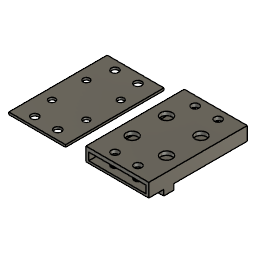
CNC Z axis (Autodesk Fusion 360 design; units mm, degrees)
part number: 2025-09-05-01-01-18-360
Autodesk Fusion 360 part; units mm, degrees
note: some values were not read from the file. Set by a fixed rule: which face or edge a step refers to.
other "Base Mesh Feature1"
other "Modify1"
sketch "Sketch1" plane through (0, 0, 0) normal (0, 0, 1) x (1, 0, 0)
  line L0 (27.5, -43) -> (-27.5, -43)
  line L1 (-27.5, -43) -> (-27.5, 43)
  line L2 (-27.5, 43) -> (27.5, 43)
  line L3 (27.5, 43) -> (27.5, -43)
  line L4 (27.5, -43) -> (-27.5, 43) construction
  line L5 (-27.5, -43) -> (27.5, 43) construction
  circle A0 centre (15, -15) radius 2.8284
  circle A1 centre (15, 15) radius 2.8284
  circle A2 centre (-15, -15) radius 2.8284
  circle A3 centre (-15, 15) radius 2.8284
  circle A4 centre (10, -35) radius 3.25
  circle A5 centre (-10, -35) radius 3.25
  circle A6 centre (10, 35) radius 3.25
  circle A7 centre (-10, 35) radius 3.25
  circle A8 centre (15, -15) radius 4.75
  circle A9 centre (15, 15) radius 4.75
  circle A10 centre (-15, -15) radius 4.75
  circle A11 centre (-15, 15) radius 4.75
  circle A12 centre (3.9244, 36.95) radius 1
  circle A13 centre (-4.0755, 36.95) radius 1
  line L6 (27.5, -21) -> (-27.5, -21)
  line L7 (27.5, 21) -> (-27.5, 21)
  line L8 (27.5, -30) -> (-27.5, -30)
  line L9 (27.5, 30) -> (-27.5, 30)
  line L10 (-6, 30) -> (-6, 43)
  line L11 (5.9128, 30) -> (5.9128, 43)
  line L12 (11.5, -30) -> (10, -29)
  line L13 (10, -29) -> (8.5, -30)
  line L14 (-8.5, -30) -> (-10, -29)
  line L15 (-10, -29) -> (-11.5, -30)
  line L16 (11.5, 30) -> (10, 29)
  line L17 (10, 29) -> (8.5, 30)
  line L18 (-8.5, 30) -> (-10, 29)
  line L19 (-10, 29) -> (-11.5, 30)
  line L20 (5.9128, 31.7978) -> (5.9175, 31.7978)
  line L21 (5.9175, 31.7978) -> (5.9175, 33.3795)
  line L22 (5.9175, 33.3795) -> (5.9128, 33.3795)
  line L23 (-6, 31.7978) -> (-6.0143, 31.7978)
  line L24 (-6.0143, 31.7978) -> (-6.0143, 33.3598)
  line L25 (-6.0143, 33.3598) -> (-6, 33.3598)
  dimension "d1" = 55
  dimension "d2" = 86
  dimension "d3" = 6.5
  dimension "d4" = 6.5
  dimension "d5" = 6.5
  dimension "d6" = 6.5
  dimension "d7" = 9.5
  dimension "d8" = 9.5
  dimension "d9" = 9.5
  dimension "d10" = 9.5
  dimension "d11" = 20
  dimension "d12" = 20
  dimension "d13" = 70
  dimension "d14" = 70
  dimension "d15" = 17.5
  dimension "d16" = 17.5
  dimension "d18" = 8
  dimension "d19" = 2
  dimension "d20" = 2
  dimension "d33" = 6.05
  dimension "d34" = 6.05
  constraint horizontal L0
  constraint perpendicular L0 L1
  constraint parallel L0 L2
  constraint parallel L1 L3
  constraint coincident L4 origin
  constraint coincident L5 origin
  constraint concentric A0 A8
  constraint concentric A1 A9
  constraint concentric A2 A10
  constraint concentric A3 A11
  constraint coincident L1 L6.end
  constraint perpendicular L1 L6
  constraint coincident L1 L7.end
  constraint perpendicular L1 L7
  constraint coincident L1 L8.end
  constraint perpendicular L1 L8
  constraint coincident L1 L9.end
  constraint perpendicular L1 L9
  constraint coincident L3 L8.start
  constraint coincident L3 L6.start
  constraint coincident L3 L7.start
  constraint coincident L3 L9.start
  constraint coincident L9 L10.start
  constraint coincident L2 L10.end
  constraint perpendicular L2 L10
  constraint coincident L9 L11.start
  constraint coincident L2 L11.end
  constraint perpendicular L2 L11
  constraint coincident L8 L12.start
  constraint coincident L8 L13.end
  constraint coincident L8 L14.start
  constraint coincident L8 L15.end
  constraint coincident L9 L16.start
  constraint parallel L15 L16
  constraint coincident L9 L17.end
  constraint parallel L14 L17
  constraint coincident L9 L18.start
  constraint parallel L16 L18
  constraint coincident L9 L19.end
  constraint parallel L17 L19
  constraint coincident L11 L20.start
  constraint perpendicular L11 L20
  constraint perpendicular L20 L21
  constraint coincident L11 L22.end
  constraint perpendicular L11 L22
  constraint coincident L10 L23.start
  constraint perpendicular L10 L23
  constraint perpendicular L23 L24
  constraint coincident L10 L25.end
  constraint perpendicular L10 L25
  measures "d1" distance of L1.end L2.end
  measures "d2" distance of L0.end L1.end
  measures "d3" diameter of A4
  measures "d4" diameter of A5
  measures "d5" diameter of A6
  measures "d6" diameter of A7
  measures "d7" diameter of A8
  measures "d8" diameter of A9
  measures "d9" diameter of A10
  measures "d10" diameter of A11
  measures "d11" distance of A4.centre A5.centre
  measures "d12" distance of A6.centre A7.centre
  measures "d13" vertical distance of A4.centre A6.centre
  measures "d14" vertical distance of A5.centre A7.centre
  measures "d15" distance of L3 A4.centre
  measures "d16" distance of L3 A6.centre
  measures "d18" distance of L0 A4.centre
  measures "d19" diameter of A12
  measures "d20" diameter of A13
  measures "d33" distance of L2 A12.centre
  measures "d34" distance of L2 A13.centre
extrude "Extrude1" add sketch "Sketch1" along normal blind 20 contours L0 L1 L3 L8 | L1 L3 L6 L8 L12 L13 L14 L15 | L1 L3 L6 L7 | L8 L12 L13 | L8 L14 L15 | L1 L3 L7 L9 L16 L17 L18 L19 | L2 L3 L9 L11 L20 L21 L22 | L1 L2 L9 L10 L23 L24 L25 | L9 L16 L17 | L9 L18 L19 | L2 L9 L10 L11 | L11 L20 L21 L22 | L10 L23 L24 L25 | A8 | A9 | A10 | A11 | A12 | A13 makes body 1
extrude "Extrude2" cut sketch "Sketch1" along normal blind 10 contours L1 L3 L6 L7 | A8 | A9 | A10 | A11 bodies 1
extrude "Extrude3" cut sketch "Sketch1" along normal blind 5 contours L1 L3 L6 L8 L12 L13 L14 L15 | L8 L12 L13 | L8 L14 L15 | L1 L3 L7 L9 L16 L17 L18 L19 | L9 L16 L17 | L9 L18 L19 bodies 1
extrude "Extrude4" cut sketch "Sketch1" along normal blind 7 contours A12 | A13 bodies 1
extrude "Extrude5" cut sketch "Sketch1" along normal blind 5 contours L0 L1 L3 L8 bodies 1
extrude "Extrude6" cut sketch "Sketch1" along normal blind 10 contours L2 L3 L9 L11 L20 L21 L22 | L1 L2 L9 L10 L23 L24 L25 | L11 L20 L21 L22 | L10 L23 L24 L25 bodies 1
sketch "Sketch2" plane through (0, 0, 0) normal (0, 0, 1) x (1, 0, 0)
extrude "Extrude7" cut sketch "Sketch1" along normal blind 10 contours L11 L20 L21 L22 | L10 L23 L24 L25 bodies 1
extrude "Extrude8" cut sketch "Sketch1" along normal blind 10 contours L9 L16 L17 | L9 L18 L19 bodies 1
extrude "Extrude9" cut sketch "Sketch1" along normal blind 10 contours L8 L12 L13 | L8 L14 L15 bodies 1
extrude "Extrude10" cut sketch "Sketch1" along normal blind 10 contours L0 L1 L3 L8 bodies 1
extrude "Extrude11" add 1 faces at (-4.3089, 4.3587, 20) along direction (0, 0, 1) blind 4 on bodies 1 bodies 1
sketch "Sketch3" plane through (0, -43, 0) normal (0, -1, 0) x (1, 0, 0)
  line L0 (-27.5, 10) -> (27.5, 10)
  line L1 (27.5, 10) -> (27.5, 24)
  line L2 (-27.5, 24) -> (-27.5, 10)
  line L3 (-26, 15.4) -> (26, 15.4)
  line L4 (26, 15.4) -> (26, 13.1)
  line L5 (26, 13.1) -> (-26, 13.1)
  line L6 (-26, 13.1) -> (-26, 15.4)
  line L7 (-26, 12.7394) -> (26, 12.7394)
  line L8 (26, 12.7394) -> (26, 10.4394)
  line L9 (26, 10.4394) -> (-26, 10.4394)
  line L10 (-26, 10.4394) -> (-26, 12.7394)
  line L11 (27.5, 24) -> (-27.5, 24)
  line L12 (-26, 18.1) -> (26, 18.1)
  line L13 (26, 18.1) -> (26, 15.8)
  line L14 (26, 15.8) -> (-26, 15.8)
  line L15 (-26, 15.8) -> (-26, 18.1)
  dimension "d61" = 2.3
  dimension "d62" = 2.3
  dimension "d65" = 2.3
  constraint horizontal L3
  constraint vertical L4
  constraint horizontal L5
  constraint vertical L6
  constraint horizontal L7
  constraint vertical L8
  constraint horizontal L9
  constraint vertical L10
  constraint horizontal L12
  constraint vertical L13
  constraint horizontal L14
  constraint vertical L15
  measures "d61" distance of L3.start L5.end
  measures "d62" distance of L7.start L9.end
  measures "d65" distance of L12.start L14.end
extrude "Extrude12" cut sketch "Sketch3" against normal blind 90 contours L3 L4 L5 L6 | L7 L8 L9 L10 bodies 1
extrude "Extrude13" add sketch "Sketch3" against normal blind 86 contours L3 L4 L5 L6 | L7 L8 L9 L10 | L12 L13 L14 L15 bodies 1
extrude "Extrude14" cut 1 faces at (-4.3089, 4.3587, 24) along direction (0, 0, -1) blind 0.6 on bodies 1 bodies 1
sketch "Sketch4" plane through (0, 0, 23.4) normal (0, 0, 1) x (-1, 0, 0)
  circle A0 centre (15, -15) radius 2.8284
  circle A1 centre (-15, 15) radius 2.8284
  circle A2 centre (-15, -15) radius 2.8284
  circle A3 centre (-10, -35) radius 3.25
  circle A4 centre (10, 35) radius 3.25
  circle A5 centre (-10, 35) radius 3.25
  circle A6 centre (15, 15) radius 2.8284
  circle A7 centre (10, -35) radius 3.25
  line L0 (-27.5, -43) -> (27.5, -43)
  line L1 (27.5, -43) -> (27.5, 43)
  line L2 (27.5, 43) -> (-27.5, 43)
  line L3 (-27.5, 43) -> (-27.5, -43)
  circle A8 centre (15, 15) radius 5
  circle A9 centre (-15, 15) radius 5
  circle A10 centre (15, -15) radius 5
  circle A11 centre (-15, -15) radius 5
  dimension "d70" = 10
  dimension "d71" = 10
  dimension "d72" = 10
  dimension "d73" = 10
  constraint concentric A6 A8
  constraint concentric A1 A9
  constraint concentric A0 A10
  constraint concentric A2 A11
  measures "d70" diameter of A8
  measures "d71" diameter of A9
  measures "d72" diameter of A10
  measures "d73" diameter of A11
extrude "Extrude15" cut sketch "Sketch4" against normal blind 6 contours A8 | A9 | A10 | A11 bodies 1
sketch "Sketch6" plane through (0, 0, 15.8) normal (0, 0, -1) x (-1, 0, 0)
  circle A0 centre (15, 15) radius 2.8284
  circle A1 centre (-15, -15) radius 2.8284
  circle A2 centre (-15, 15) radius 2.8284
  circle A3 centre (-10, 35) radius 3.25
  circle A4 centre (10, -35) radius 3.25
  circle A5 centre (-10, -35) radius 3.25
  circle A6 centre (15, -15) radius 2.8284
  circle A7 centre (10, 35) radius 3.25
extrude "Extrude17" add 1 faces at (5.9128, 38.6667, 5) along direction (1, 0, 0) blind 1 on bodies 1 bodies 1
extrude "Extrude18" add 1 faces at (-6, 38.6667, 5) along direction (-1, 0, 0) blind 1 on bodies 1 bodies 1
sketch "Sketch7" plane through (0, -43, 0) normal (0, -1, 0) x (1, 0, 0)
  line L0 (27.5, 23.4) -> (-27.5, 23.4)
  line L1 (-27.5, 23.4) -> (-27.5, 10)
  line L2 (-27.5, 10) -> (27.5, 10)
  line L3 (27.5, 10) -> (27.5, 23.4)
  line L4 (-25, 20.1) -> (25, 20.1)
  line L5 (25, 20.1) -> (25, 12)
  line L6 (25, 12) -> (-25, 12)
  line L7 (-25, 12) -> (-25, 20.1)
  dimension "d82" = 2.5
  dimension "d83" = 2.5
  dimension "d84" = 3.3
  dimension "d85" = 2
  constraint horizontal L4
  constraint vertical L5
  constraint horizontal L6
  constraint vertical L7
  measures "d82" distance of L3 L5
  measures "d83" distance of L1 L7
  measures "d84" distance of L0 L4
  measures "d85" distance of L2 L6
extrude "Extrude19" cut sketch "Sketch7" against normal blind 100 contours L4 L5 L6 L7 bodies 1
extrude "Extrude20" cut 8 faces at (-9.7589, -36.0562, 10.4394) (9.1107, -33.6316, 10.4394) (15.6184, -15.9402, 10.4394) (-14.1276, -14.0598, 10.4394) (-14.5286, 13.6277, 10.4394) (15.779, 15.5311, 10.4394) (10.7036, 35.9382, 10.4394) (-11.0184, 36.0101, 10.4394) along direction (0, 0, 1) blind 8 on bodies 1 bodies 1
sketch "Sketch8" plane through (0, 0, 0) normal (0, 0, 1) x (1, 0, 0)
sketch "Sketch9" plane through (6.9128, 0, 0) normal (1, 0, 0) x (0, 1, 0)
  line L0 (30, 0) -> (43, 0)
  line L1 (43, 0) -> (43, 10)
  line L2 (43, 10) -> (36.0156, 10)
  line L3 (36.0156, 10) -> (33.9844, 10)
  line L4 (33.9844, 10) -> (30, 10)
  line L5 (30, 10) -> (30, 5)
  line L6 (30, 5) -> (30, 0)
  line L7 (31.5, 10) -> (40, 10)
  line L8 (40, 10) -> (40, 4.9746)
  line L9 (40, 4.9746) -> (31.5, 4.9746)
  line L10 (31.5, 4.9746) -> (31.5, 10)
  dimension "d94" = 1.5
  dimension "d95" = 3
  constraint horizontal L7
  constraint vertical L8
  constraint horizontal L9
  constraint vertical L10
  constraint coincident L4 L7.start
  measures "d94" distance of L6 L10
  measures "d95" distance of L1 L8
extrude "Extrude21" cut sketch "Sketch9" against normal blind 2 contours L2 L3 L4 L7 L8 L9 L10 bodies 1
sketch "Sketch10" plane through (-7, 0, 0) normal (-1, 0, 0) x (0, -1, 0)
  line L0 (-43, 0) -> (-30, 0)
  line L1 (-30, 0) -> (-30, 5)
  line L2 (-30, 5) -> (-30, 10)
  line L3 (-30, 10) -> (-33.75, 10)
  line L4 (-33.75, 10) -> (-36.25, 10)
  line L5 (-36.25, 10) -> (-43, 10)
  line L6 (-43, 10) -> (-43, 0)
  line L7 (-31.5, 10) -> (-40, 10)
  line L8 (-40, 10) -> (-40, 5)
  line L9 (-40, 5) -> (-31.5, 5)
  line L10 (-31.5, 5) -> (-31.5, 10)
  constraint horizontal L7
  constraint vertical L8
  constraint horizontal L9
  constraint vertical L10
  constraint coincident L3 L7.start
extrude "Extrude22" cut sketch "Sketch10" against normal blind 3.5 contours L3 L4 L5 L7 L8 L9 L10 bodies 1
sketch "Sketch12" plane through (0, 0, 12) normal (0, 0, 1) x (-1, 0, 0)
  circle A0 centre (-10, -35) radius 3.25
  circle A1 centre (15, -15) radius 2.8284
  circle A2 centre (-15, 15) radius 2.8284
  circle A3 centre (10, 35) radius 3.25
  circle A4 centre (-10, 35) radius 3.25
  circle A5 centre (15, 15) radius 2.8284
  circle A6 centre (-15, -15) radius 2.8284
  circle A7 centre (10, -35) radius 3.25
  line L0 (-25, -43) -> (25, -43)
  line L1 (25, -43) -> (25, 43)
  line L2 (25, 43) -> (-25, 43)
  line L3 (-25, 43) -> (-25, -43)
extrude "Extrude23" add 1 faces at (4.3089, -4.3587, 12) along direction (0, 0, 1) blind 2 separate body on bodies 1 makes body 2
move_body "Move2" bodies 2 to x (1, 0, 0) y (0, 1, 0) z (0, 0, 1) at (-70, 0, 0)
sketch "Sketch13" plane through (0, 0, 14) normal (0, 0, 1) x (-1, 0, 0)
  circle A0 centre (60, -35) radius 3.25
  circle A1 centre (85, -15) radius 2.8284
  circle A2 centre (55, 15) radius 2.8284
  circle A3 centre (80, 35) radius 3.25
  circle A4 centre (60, 35) radius 3.25
  circle A5 centre (85, 15) radius 2.8284
  circle A6 centre (55, -15) radius 2.8284
  circle A7 centre (80, -35) radius 3.25
  line L0 (45, -43) -> (95, -43)
  line L1 (95, -43) -> (95, 43)
  line L2 (95, 43) -> (45, 43)
  line L3 (45, 43) -> (45, -43)
  line L4 (94.8, 43) -> (94.8, -43)
  line L5 (45.2, 43) -> (45.2, -43)
  dimension "d98" = 0.2
  dimension "d99" = 0.2
  constraint coincident L2 L4.start
  constraint coincident L0 L4.end
  constraint perpendicular L0 L4
  constraint coincident L2 L5.start
  constraint coincident L0 L5.end
  constraint perpendicular L0 L5
  measures "d98" distance of L1 L4
  measures "d99" distance of L3 L5
extrude "Extrude24" cut sketch "Sketch13" against normal blind 10 contours L0 L1 L2 L4 bodies 2
extrude "Extrude25" cut sketch "Sketch13" against normal blind 5 contours L0 L2 L3 L5 bodies 2
extrude "Extrude26" cut 1 faces at (-5.8333, 31.5, 6.6667) along direction (0, -1, 0) blind 1.5 on bodies 1 bodies 1
extrude "Extrude27" add 1 faces at (-3.5, 32.5441, 7.3333) along direction (-1, 0, 0) blind 0.5 on bodies 1 bodies 1
extrude "Extrude28" cut 1 faces at (4.9128, 33.266, 7.3249) along direction (-1, 0, 0) blind 1.5 on bodies 1 bodies 1
extrude "Extrude29" cut 2 faces at (6.2461, 31.5, 6.6498) (4.4128, 31.5, 6.6498) along direction (0, -1, 0) blind 1.5 on bodies 1 bodies 1
extrude "Extrude30" add 2 faces at (3.4128, 31, 6.6582) (3.4128, 33.0303, 7.3249) along direction (1, 0, 0) blind 0.5 on bodies 1 bodies 1
extrude "Extrude31" add 1 faces at (-3.7782, -3.8664, 20.1) along direction (0, 0, -1) blind 1.5 on bodies 1 bodies 1
extrude "Extrude32" cut 1 faces at (3.7782, -3.8664, 23.4) along direction (0, 0, -1) blind 1.5 on bodies 1 bodies 1
sketch "Sketch14" plane through (0, 0, 5) normal (0, 0, -1) x (1, 0, 0)
  line L0 (10, -29) -> (11.5, -30)
  line L1 (11.5, -30) -> (27.5, -30)
  line L2 (27.5, -30) -> (27.5, -21)
  line L3 (27.5, -21) -> (-27.5, -21)
  line L4 (-27.5, -21) -> (-27.5, -30)
  line L5 (-27.5, -30) -> (-11.5, -30)
  line L6 (-11.5, -30) -> (-10, -29)
  line L7 (-10, -29) -> (-8.5, -30)
  line L8 (-8.5, -30) -> (-7, -30)
  line L9 (-7, -30) -> (-4, -30)
  line L10 (-4, -30) -> (3.9128, -30)
  line L11 (3.9128, -30) -> (8.5, -30)
  line L12 (8.5, -30) -> (10, -29)
  line L13 (-7.5, -30) -> (-7.5, -21)
  line L14 (7.4128, -30) -> (7.4128, -21)
  line L15 (-7, -43) -> (-7, -30)
  line L16 (6.9128, -30) -> (6.9128, -43)
  line L17 (-7.5, -30) -> (-27.5, -30)
  line L18 (-27.5, -30) -> (-27.5, -21)
  line L19 (-27.5, -21) -> (-7.5, -21)
  line L20 (-7.5, -21) -> (-7.5, -30)
  line L21 (7.4128, -30) -> (27.5, -30)
  line L22 (27.5, -30) -> (27.5, -21)
  line L23 (27.5, -21) -> (7.4128, -21)
  line L24 (7.4128, -21) -> (7.4128, -30)
  dimension "d118" = 0.5
  dimension "d119" = 0.5
  constraint coincident L8 L13.start
  constraint coincident L3 L13.end
  constraint perpendicular L3 L13
  constraint coincident L11 L14.start
  constraint coincident L3 L14.end
  constraint perpendicular L3 L14
  constraint horizontal L17
  constraint vertical L18
  constraint horizontal L19
  constraint vertical L20
  constraint coincident L3.end L4.start
  constraint horizontal L21
  constraint vertical L22
  constraint horizontal L23
  constraint vertical L24
  constraint coincident L2.end L3.start
  measures "d118" distance of L13.start L15
  measures "d119" distance of L14.start L16
extrude "Extrude33" cut sketch "Sketch14" against normal blind 5 contours L3 L4 L5 L6 L7 L8 L13 L17 L18 L19 L20 bodies 1
sketch "Sketch15" plane through (0, 0, 5) normal (0, 0, -1) x (1, 0, 0)
  line L0 (-7.5, -21) -> (-7.5, -30)
  line L1 (-7.5, -30) -> (-7, -30)
  line L2 (-7, -30) -> (-4, -30)
  line L3 (-4, -30) -> (3.9128, -30)
  line L4 (3.9128, -30) -> (8.5, -30)
  line L5 (8.5, -30) -> (10, -29)
  line L6 (10, -29) -> (11.5, -30)
  line L7 (11.5, -30) -> (27.5, -30)
  line L8 (27.5, -30) -> (27.5, -21)
  line L9 (27.5, -21) -> (-7.5, -21)
sketch "Sketch16" plane through (0, 0, 0) normal (0, 0, 1) x (1, 0, 0)
  line L0 (7.4128, 30) -> (7.4128, 21)
  line L1 (6.9128, 30) -> (6.9128, 43)
  line L2 (7.4128, 21) -> (27.4789, 21)
  line L3 (27.4789, 21) -> (27.4789, 30)
  line L4 (27.4789, 30) -> (7.4128, 30)
  line L5 (7.4128, 30) -> (7.4128, 21)
  dimension "d122" = 0.5
  constraint vertical L0
  constraint horizontal L2
  constraint vertical L3
  constraint horizontal L4
  constraint vertical L5
  measures "d122" distance of L0.start L1
extrude "Extrude34" cut sketch "Sketch16" along normal blind 10 bodies 1
delete_face "DeleteFace1" 1 faces at (27.4789, 24, 6.6667) on bodies 1
